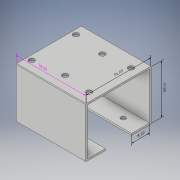
# Autodesk Inventor part: suport motor
Saved by Autodesk Inventor 2019 (Build 230136000, 136)
## iProperties
Created: 2018-08-07
Part Number: suport motor
Material: Genérico
Document SubType Name: Modeling
Designer: Albert Garangou Culebras
Density: 1 g/cm^3
Appearance: Valor por defecto
Author: Albert Garangou Culebras
Autodesk Inventor part; units mm, degrees
ref_plane "YZ Plane" through (0, 0, 0) normal (1, 0, 0) x (0, 1, 0)
ref_plane "XZ Plane" through (0, 0, 0) normal (0, 1, 0) x (-1, 0, 0)
ref_plane "XY Plane" through (0, 0, 0) normal (0, 0, 1) x (1, 0, 0)
sketch "Boceto1" plane through (0, 0, 0) normal (0, 1, 0) x (-1, 0, 0)
  line L0 (0, 0) -> (-58, 0)
  line L1 (-58, 0) -> (-58, -55)
  line L2 (-58, -55) -> (0, -55)
  line L3 (0, -55) -> (0, 0)
  line L4 (0, -55) -> (-58, -55)
  dimension "d0" = 58
  dimension "d1" = 55
  constraints: 10 end point, 2 horizontal, 2 parallel, 1 perpendicular
  measures "d0" distance of L2.end L1.end
  measures "d1" distance of L1.end L0.end
extrude "Extrusión1" add sketch "Boceto1" along normal blind 1.5
sketch "Boceto3" plane through (0, 0, 0) normal (0, 0, 1) x (1, 0, 0)
  line L0 (0, 1.5) -> (58, 1.5) projected
  line L1 (58, 1.5) -> (0, 1.5)
  line L2 (0, 1.5) -> (0, -40.5)
  line L3 (0, -40.5) -> (58, -40.5)
  line L4 (58, -40.5) -> (58, 1.5)
  point P0 (0, 0)
  dimension "d8" = 58
  dimension "d9" = 42
  constraints: 8 end point, 2 parallel, 1 horizontal, 1 perpendicular
  measures "d8" distance of L3.end L2.end
  measures "d9" distance of L2.end L1.end
sketch "Boceto4" plane through (58, 0, -55) normal (0, 0, -1) x (-1, 0, 0)
  line L0 (58, 1.5) -> (0, 1.5) projected
  line L1 (0, 1.5) -> (58, 1.5)
  line L2 (58, 1.5) -> (58, -40.5)
  line L3 (58, -40.5) -> (0, -40.5)
  line L4 (0, -40.5) -> (0, 1.5)
  point P0 (58, 0)
  dimension "d10" = 42
  constraints: 8 end point, 2 parallel, 1 horizontal, 1 perpendicular
  measures "d10" distance of L1.end L2.end
extrude "Extrusión2" add sketch "Boceto4" against normal blind 1.5
extrude "Extrusión3" add sketch "Boceto3" against normal blind 1.5
sketch "Boceto6" plane through (0, -40.5, 0) normal (0, -1, 0) x (1, 0, 0)
  line L0 (58, 0) -> (58, -1.5) projected
  line L1 (58, -1.5) -> (0, -1.5)
  line L2 (58, -1.5) -> (0, -1.5)
  line L3 (0, -1.5) -> (0, -16.5)
  line L4 (0, -16.5) -> (58, -16.5)
  line L5 (58, -16.5) -> (58, -1.5)
  line L6 (58, -55) -> (0, -55)
  line L7 (58, -40) -> (58, -55)
  line L8 (0, -53.5) -> (58, -53.5)
  line L9 (58, -53.5) -> (58, -38.5)
  line L10 (58, -38.5) -> (0, -38.5)
  line L11 (0, -38.5) -> (0, -53.5)
  point P0 (0, 0)
  dimension "d17" = 15
  dimension "d50" = 15
  dimension "d51" = 58
  dimension "d61" = 58
  dimension "d62" = 15
  constraints: 22 end point, 4 horizontal, 4 parallel, 2 perpendicular, 1 point on line
  measures "d17" distance of L3.end L2.end
  measures "d50" distance of L4.end L0.end
  measures "d51" distance of L3.end L4.end
  measures "d61" distance of L10.end L9.end
  measures "d62" distance of L9.end L8.end
extrude "Extrusión4" add sketch "Boceto6" against normal blind 1.5
sketch "Boceto7" plane through (0, -40.5, 0) normal (0, -1, 0) x (1, 0, 0)
  line L0 (58, 0) -> (58, -16.5) projected
  line L1 (0, 0) -> (0, -16.5) projected
  line L2 (58, -55) -> (58, -38.5) projected
  circle A0 centre (43.5, -8.25) radius 2
  circle A1 centre (14.5, -8.25) radius 2
  line L3 (0, -53.5) -> (0, -38.5) projected
  line L4 (0, -46) -> (58, -46)
  line L5 (58, -38.5) -> (58, -53.5) projected
  circle A2 centre (43.5, -46) radius 2
  circle A3 centre (14.5, -46) radius 2
  point P0 (58, -40)
  dimension "d23" = 4
  dimension "d25" = 4
  dimension "d63" = 4
  dimension "d64" = 4
  constraints: 4 centre point, 2 end point, 2 midpoint, 2 point on line
  measures "d23" diameter of A0
  measures "d25" diameter of A1
  measures "d63" diameter of A2
  measures "d64" diameter of A3
extrude "Extrusión5" cut sketch "Boceto7" against normal blind 1.5
sketch "Boceto8" plane through (0, 1.5, 0) normal (0, 1, 0) x (1, 0, 0)
  line L0 (58, 0) -> (58, 55) projected
  line L1 (58, 1.5) -> (58, 53.5) projected
  line L2 (58, 45) -> (51, 45)
  circle A0 centre (51, 45) radius 2.25
  circle A1 centre (51, 10) radius 2.25
  circle A2 centre (4, 9) radius 2.25
  circle A3 centre (4, 46) radius 2.25
  circle A4 centre (29, 12) radius 2.25
  circle A5 centre (29, 43) radius 2.25
  point P0 (0, 0)
  point P1 (0, 55)
  dimension "d32" = 7
  dimension "d33" = 4.5
  dimension "d34" = 4.5
  dimension "d39" = 4.5
  dimension "d40" = 4.5
  dimension "d45" = 4.5
  dimension "d47" = 4.5
  constraints: 6 centre point, 2 end point, 1 coincident, 1 point on line
  measures "d32" distance of L2.start L2.end
  measures "d33" diameter of A0
  measures "d34" diameter of A1
  measures "d39" diameter of A2
  measures "d40" diameter of A3
  measures "d45" diameter of A4
  measures "d47" diameter of A5
extrude "Extrusión7" cut sketch "Boceto8" against normal blind 1.5
fillet "Empalme1" radius 0.5 4 edges at (29, 1.5, -55) (29, -40.5, -55) (29, -40.5, 0) (29, 1.5, 0)
